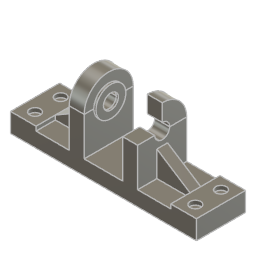
viking (Autodesk Fusion 360 design; units mm, degrees)
Autodesk Fusion 360 part; units mm, degrees
note: some values were not read from the file. Set by a fixed rule: which sketch regions a step uses.
sketch "Sketch1" plane through (0, 0, 0) normal (0, 1, 0) x (1, 0, 0)
  line L0 (0, 0) -> (87, 0)
  line L1 (0, 0) -> (-87, 0)
  line L2 (-87, 0) -> (-87, 46)
  line L3 (87, 0) -> (87, 46)
  line L4 (-87, 46) -> (87, 46)
  dimension "d1" = 87
  dimension "d2" = 87
  dimension "d3" = 46
  dimension "d4" = 46
  constraint coincident L0.start L1.start
  constraint horizontal L0
  constraint parallel L0 L1
  constraint perpendicular L1 L2
  constraint perpendicular L0 L3
  measures "d1" distance of L0.start L0.end
  measures "d2" distance of L0.start L1.end
  measures "d3" distance of L1.end L2.end
  measures "d4" distance of L0.end L3.end
extrude "Extrude1" add sketch "Sketch1" along normal blind 14 makes body 1
sketch "Sketch2" plane through (0, 14, 0) normal (0, 1, 0) x (-1, 0, 0)
  line L0 (87, 0) -> (-87, 0)
  line L1 (-87, 0) -> (-87, -46)
  line L2 (-87, -46) -> (87, -46)
  line L3 (87, -46) -> (87, 0)
  line L4 (87, -46) -> (-87, -46)
  line L5 (-87, -46) -> (-87, 0)
  line L6 (-87, 0) -> (87, 0)
  line L7 (87, 0) -> (87, -46)
  line L8 (-87, -46) -> (-63, -46)
  line L9 (-63, -46) -> (-63, 0)
  line L10 (-63, 0) -> (-87, 0)
  line L11 (-87, 0) -> (-87, -46)
  line L12 (87, -46) -> (63, -46)
  line L13 (63, -46) -> (63, 0)
  line L14 (63, 0) -> (87, 0)
  line L15 (87, 0) -> (87, -46)
  line L16 (87, -46) -> (87, -23) construction
  line L17 (87, -23) -> (-87, -23) construction
  line L18 (87, -23) -> (87, -11) construction
  line L19 (87, -23) -> (87, -35) construction
  line L20 (87, -35) -> (-87, -35) construction
  line L21 (87, -11) -> (-87, -11) construction
  line L22 (87, -46) -> (75, -46) construction
  line L23 (75, -46) -> (75, 0) construction
  line L24 (-63, -46) -> (-75, -46) construction
  line L25 (-75, -46) -> (-75, 0) construction
  circle A0 centre (75, -35) radius 5
  circle A1 centre (75, -11) radius 5
  circle A2 centre (-75, -35) radius 5
  circle A3 centre (-75, -11) radius 5
  dimension "d7" = 24
  dimension "d8" = 24
  dimension "d9" = 46
  dimension "d10" = 12
  dimension "d11" = 12
  dimension "d12" = 10
  dimension "d13" = 10
  dimension "d14" = 10
  dimension "d15" = 10
  constraint horizontal L4
  constraint vertical L5
  constraint horizontal L6
  constraint vertical L7
  constraint coincident L0.end L1.start
  constraint coincident L2.end L3.start
  constraint horizontal L8
  constraint vertical L9
  constraint horizontal L10
  constraint vertical L11
  constraint coincident L6 L9.end
  constraint coincident L1.end L2.start
  constraint horizontal L12
  constraint vertical L13
  constraint horizontal L14
  constraint vertical L15
  constraint midpoint L3 L16.end
  constraint midpoint L11 L17.end
  constraint perpendicular L17 L18
  constraint perpendicular L17 L19
  constraint coincident L5 L20.end
  constraint perpendicular L5 L20
  constraint coincident L1 L21.end
  constraint perpendicular L1 L21
  constraint midpoint L12 L22.end
  constraint midpoint L14 L23.end
  constraint midpoint L8 L24.end
  constraint midpoint L10 L25.end
  constraint coincident L20 A0.centre
  constraint coincident L23 A0.centre
  constraint coincident L21 A1.centre
  constraint coincident L23 A1.centre
  constraint coincident L25 A2.centre
  constraint coincident L20 A2.centre
  constraint coincident L21 A3.centre
  constraint coincident L25 A3.centre
  measures "d7" distance of L1.end L8.end
  measures "d8" distance of L2.end L12.end
  measures "d9" distance of L2.end L0.start
  measures "d10" distance of L16.end L18.end
  measures "d11" distance of L16.end L19.end
  measures "d12" diameter of A0
  measures "d13" diameter of A1
  measures "d14" diameter of A2
  measures "d15" diameter of A3
extrude "Extrude2" add sketch "Sketch2" along normal blind 4 contours L0 L2 L3 L4 L6 L7 L12 L13 L14 L15 bodies 1
extrude "Extrude3" add sketch "Sketch2" along normal blind 4 contours L0 L1 L2 L4 L5 L6 L8 L9 L10 L11 bodies 1
sketch "Sketch3" plane through (0, 0, 0) normal (0, 0, 1) x (1, 0, 0)
  line L0 (-87, 0) -> (87, 0)
  line L1 (87, 0) -> (87, 18)
  line L2 (87, 18) -> (63, 18)
  line L3 (63, 18) -> (63, 14)
  line L4 (63, 14) -> (-63, 14)
  line L5 (-63, 14) -> (-63, 18)
  line L6 (-63, 18) -> (-87, 18)
  line L7 (-87, 18) -> (-87, 0)
  line L8 (0, 0) -> (-75, 0) construction
  line L9 (-75, 0) -> (-75, 18) construction
  line L10 (75, 18) -> (75, 0) construction
  line L11 (75, 0) -> (-75, 0) construction
  line L12 (87, 0) -> (32, 0) construction
  line L13 (0, 0) -> (75, 0) construction
  line L14 (32, 0) -> (32, 50) construction
  line L15 (32, 14) -> (32, 50)
  line L16 (32, 50) -> (18, 50)
  line L17 (18, 50) -> (18, 14)
  line L18 (32, 14) -> (-32, 14) construction
  line L19 (-32, 14) -> (-32, 50)
  line L20 (-32, 50) -> (-18, 50)
  line L21 (-18, 50) -> (-18, 14)
  dimension "d20" = 75
  dimension "d21" = 55
  dimension "d22" = 50
  dimension "d23" = 14
  dimension "d24" = 64
  dimension "d25" = 14
  constraint coincident L8.start L13.start
  constraint perpendicular L3 L8
  constraint midpoint L6 L9.end
  constraint coincident L0 L10.end
  constraint perpendicular L0 L10
  constraint coincident L0.end L1.start
  constraint perpendicular L1 L12
  constraint perpendicular L13 L14
  constraint coincident L4 L15.start
  constraint coincident L14 L15.start
  constraint perpendicular L14 L16
  constraint coincident L4 L17.end
  constraint perpendicular L4 L17
  constraint perpendicular L17 L18
  constraint perpendicular L18 L19
  constraint perpendicular L19 L20
  constraint coincident L18 L21.end
  measures "d20" distance of L8.start L8.end
  measures "d21" distance of L0.end L12.end
  measures "d22" distance of L12.end L14.end
  measures "d23" distance of L14.end L16.end
  measures "d24" distance of L15.start L18.end
  measures "d25" distance of L19.end L20.end
extrude "Extrude4" add sketch "Sketch3" against normal blind 46 contours L4 L15 L16 L17 bodies 1
extrude "Extrude5" add sketch "Sketch3" against normal blind 46 contours L4 L19 L20 L21 bodies 1
sketch "Sketch4" plane through (-18, 0, 0) normal (1, 0, 0) x (0, 0, -1)
  line L0 (0, 50) -> (0, 14)
  line L1 (0, 14) -> (46, 14)
  line L2 (46, 14) -> (46, 50)
  line L3 (46, 50) -> (0, 50)
  line L4 (0, 50) -> (0, 18)
  line L5 (0, 18) -> (46, 18)
  line L6 (46, 18) -> (46, 50)
  line L7 (46, 50) -> (0, 50)
  circle A0 centre (23, 50) radius 14
  circle A1 centre (23, 50) radius 7
  arc A2 (46, 50) -> (0, 50) centre (23, 50) ccw
  line L8 (0, 50) -> (0, 18)
  line L9 (0, 18) -> (46, 18)
  line L10 (46, 18) -> (46, 50)
  dimension "d30" = 28
  dimension "d31" = 14
  constraint coincident L0.start L3.end
  constraint coincident L0 L4.end
  constraint perpendicular L1 L4
  constraint coincident L2 L5.end
  constraint perpendicular L2 L5
  constraint coincident L2.end L3.start
  constraint perpendicular L3 L6
  constraint midpoint L7 A0.centre
  constraint coincident L2.end A2
  constraint concentric A0 A2
  constraint concentric A0 A1
  constraint perpendicular L5 L8
  measures "d30" diameter of A0
  measures "d31" diameter of A1
extrude "Extrude6" add sketch "Sketch4" against normal blind 14 contours L3 L7 A0 A2 bodies 1
extrude "Extrude7" add sketch "Sketch4" along normal blind 2 separate body contours L3 L7 A0 A1 picked at (29.4096, 59.7107) makes body 2
extrude "Extrude8" add sketch "Sketch4" along normal blind 2 contours L3 L7 A0 A1 picked at (11.4115, 48.9567) bodies 1 2
sketch "Sketch5" plane through (-32, 0, 0) normal (-1, 0, 0) x (0, 0, 1)
  line L0 (-9, 50) -> (-37, 50)
  arc A0 (-9, 50) -> (-37, 50) centre (-23, 50) ccw
  arc A1 (0, 50) -> (-46, 50) centre (-23, 50) ccw
  line L1 (-46, 50) -> (-46, 14)
  line L2 (-46, 14) -> (0, 14)
  line L3 (0, 14) -> (0, 50)
  circle A2 centre (-23, 50) radius 14
  circle A3 centre (-23, 50) radius 7
  arc A4 (0, 50) -> (-46, 50) centre (-23, 50) ccw
  dimension "d38" = 46
  dimension "d39" = 28
  dimension "d40" = 14
  constraint concentric A0 A4
  constraint concentric A2 A4
  constraint concentric A3 A4
  measures "d38" diameter of A4
  measures "d39" diameter of A2
  measures "d40" diameter of A3
extrude "Extrude9" add sketch "Sketch5" along normal blind 2 separate body contours L0 A2 A3 | L0 A0 A2 A3 makes body 3
sketch "Sketch6" plane through (32, 0, 0) normal (1, 0, 0) x (0, 0, -1)
  line L0 (0, 50) -> (0, 14)
  line L1 (0, 14) -> (46, 14)
  line L2 (46, 14) -> (46, 50)
  line L3 (46, 50) -> (0, 50)
  circle A0 centre (23, 50) radius 7
  line L4 (23, 57) -> (23, 73)
  line L5 (9, 50) -> (0, 50)
  line L6 (9, 50) -> (0, 50)
  arc A1 (46, 50) -> (0, 50) centre (23, 50) ccw
  dimension "d43" = 14
  dimension "d45" = 46
  constraint midpoint L3 A0.centre
  constraint concentric A0 A1
  constraint coincident A0 L4.start
  constraint coincident L4.end A1
  constraint vertical L4
  constraint coincident L3 L5.start
  constraint coincident L0.start L3.end
  measures "d43" diameter of A0
  measures "d45" diameter of A1
extrude "Extrude10" add sketch "Sketch6" against normal blind 14 separate body contours L3 A0 L4 A1 makes body 4
extrude "Extrude11" cut sketch "Sketch6" against normal blind 14 contours L3 A0 picked at (23.8525, 47.828) bodies 1
sketch "Sketch7" plane through (0, 0, 0) normal (0, 0, 1) x (1, 0, 0)
  line L0 (-87, 0) -> (87, 0)
  line L1 (87, 0) -> (87, 18)
  line L2 (87, 18) -> (63, 18)
  line L3 (63, 18) -> (63, 14)
  line L4 (63, 14) -> (32, 14)
  line L5 (32, 14) -> (32, 50)
  line L6 (32, 50) -> (18, 50)
  line L7 (18, 50) -> (18, 14)
  line L8 (18, 14) -> (-18, 14)
  line L9 (-18, 14) -> (-18, 50)
  line L10 (-18, 50) -> (-32, 50)
  line L11 (-32, 50) -> (-32, 14)
  line L12 (-32, 14) -> (-63, 14)
  line L13 (-63, 14) -> (-63, 18)
  line L14 (-63, 18) -> (-87, 18)
  line L15 (-87, 18) -> (-87, 0)
  line L16 (32, 50) -> (32, 38)
  line L17 (32, 38) -> (63, 18)
  line L18 (32, 38) -> (32, 14)
  line L19 (32, 14) -> (63, 14)
  line L20 (63, 14) -> (63, 10)
  line L21 (-32, 36) -> (-63, 18)
  line L22 (-63, 18) -> (-63, 14)
  line L23 (-63, 14) -> (-32, 14)
  line L24 (-32, 14) -> (-32, 36)
  dimension "d50" = 12
  constraint coincident L5.end L6.start
  constraint perpendicular L6 L16
  constraint coincident L2.end L3.start
  constraint coincident L4.end L5.start
  constraint coincident L3.end L4.start
  constraint perpendicular L2 L20
  constraint coincident L11 L21.start
  constraint coincident L13.end L14.start
  constraint coincident L12.end L13.start
  constraint coincident L11.end L12.start
  measures "d50" distance of L5.end L16.end
sketch "Sketch8" plane through (0, 0, -46) normal (0, 0, -1) x (-1, 0, 0)
  line L0 (-87, 0) -> (87, 0)
  line L1 (87, 0) -> (87, 18)
  line L2 (87, 18) -> (63, 18)
  line L3 (63, 18) -> (63, 14)
  line L4 (63, 14) -> (32, 14)
  line L5 (32, 14) -> (32, 50)
  line L6 (32, 50) -> (18, 50)
  line L7 (18, 50) -> (18, 14)
  line L8 (18, 14) -> (-18, 14)
  line L9 (-18, 14) -> (-18, 50)
  line L10 (-18, 50) -> (-32, 50)
  line L11 (-32, 50) -> (-32, 14)
  line L12 (-32, 14) -> (-63, 14)
  line L13 (-63, 14) -> (-63, 18)
  line L14 (-63, 18) -> (-87, 18)
  line L15 (-87, 18) -> (-87, 0)
  line L16 (-63, 18) -> (-32, 38)
  line L17 (-32, 38) -> (-32, 14)
  line L18 (-32, 14) -> (-63, 14)
  line L19 (63, 18) -> (32, 36)
  line L20 (32, 36) -> (32, 14)
  line L21 (32, 14) -> (63, 14)
  line L22 (63, 14) -> (63, 18)
  constraint coincident L13.end L14.start
  constraint coincident L11 L16.end
  constraint coincident L11.end L12.start
  constraint coincident L12.end L13.start
  constraint coincident L2.end L3.start
  constraint coincident L5 L19.end
  constraint coincident L4.end L5.start
  constraint coincident L3.end L4.start
extrude "Extrude12" add sketch "Sketch7" against normal blind 18 separate body contours L3 L4 L5 L17 L18 L19 makes body 5
extrude "Extrude13" add sketch "Sketch8" against normal blind 18 separate body contours L11 L12 L13 L16 L17 L18 makes body 6
extrude "Extrude14" add 1 faces at (42.3333, 23.3333, -18) along direction (0, 0, -1) blind 10 on bodies 5 bodies 1 3 4 5 6
sketch "Sketch9" plane through (0, 0, 0) normal (0, 0, 1) x (1, 0, 0)
  line L0 (-87, 0) -> (87, 0)
  line L1 (87, 0) -> (87, 18)
  line L2 (87, 18) -> (63, 18)
  line L3 (63, 18) -> (32, 38)
  line L4 (32, 38) -> (32, 50)
  line L5 (32, 50) -> (18, 50)
  line L6 (18, 50) -> (18, 14)
  line L7 (18, 14) -> (-18, 14)
  line L8 (-18, 14) -> (-18, 50)
  line L9 (-18, 50) -> (-32, 50)
  line L10 (-32, 50) -> (-32, 14)
  line L11 (-32, 14) -> (-63, 14)
  line L12 (-63, 14) -> (-63, 18)
  line L13 (-63, 18) -> (-87, 18)
  line L14 (-87, 18) -> (-87, 0)
  line L15 (32, 38) -> (32, 14)
  line L16 (32, 14) -> (63, 14)
  line L17 (63, 14) -> (63, 18)
  constraint coincident L3.end L4.start
  constraint parallel L4 L15
  constraint perpendicular L15 L16
  constraint coincident L2.end L3.start
extrude "Extrude15" cut sketch "Sketch9" against normal blind 18 contours L3 L15 L16 L17 bodies 1
sketch "Sketch10" plane through (0, 0, -46) normal (0, 0, -1) x (-1, 0, 0)
  line L0 (-87, 0) -> (87, 0)
  line L1 (87, 0) -> (87, 18)
  line L2 (87, 18) -> (63, 18)
  line L3 (63, 18) -> (63, 14)
  line L4 (63, 14) -> (32, 14)
  line L5 (32, 14) -> (32, 50)
  line L6 (32, 50) -> (18, 50)
  line L7 (18, 50) -> (18, 14)
  line L8 (18, 14) -> (-18, 14)
  line L9 (-18, 14) -> (-18, 50)
  line L10 (-18, 50) -> (-32, 50)
  line L11 (-32, 50) -> (-32, 38)
  line L12 (-32, 38) -> (-63, 18)
  line L13 (-63, 18) -> (-87, 18)
  line L14 (-87, 18) -> (-87, 0)
  line L15 (-63, 14) -> (-63, 18)
  line L16 (-63, 14) -> (-32, 14)
  line L17 (-32, 14) -> (-32, 39)
  line L18 (-63, 18) -> (-32, 38)
  constraint coincident L12.end L13.start
  constraint perpendicular L13 L15
  constraint perpendicular L9 L16
  constraint perpendicular L8 L17
  constraint coincident L11.end L12.start
extrude "Extrude16" cut sketch "Sketch10" against normal blind 18 contours L12 L15 L16 L17 L18 bodies 1
sketch "Sketch11" plane through (0, 0, 0) normal (0, 0, 1) x (1, 0, 0)
  line L0 (32, 14) -> (32, 50)
  line L1 (32, 50) -> (18, 50)
  line L2 (18, 50) -> (18, 14)
  line L3 (18, 14) -> (-18, 14)
  line L4 (-18, 14) -> (-18, 50)
  line L5 (-18, 50) -> (-32, 50)
  line L6 (-32, 50) -> (-32, 14)
  line L7 (-32, 14) -> (-63, 14)
  line L8 (-63, 14) -> (-63, 18)
  line L9 (-63, 18) -> (-87, 18)
  line L10 (-87, 18) -> (-87, 0)
  line L11 (-87, 0) -> (87, 0)
  line L12 (87, 0) -> (87, 18)
  line L13 (87, 18) -> (63, 18)
  line L14 (63, 18) -> (63, 14)
  line L15 (63, 14) -> (32, 14)
  line L16 (-63, 18) -> (-32, 36)
  line L17 (-32, 36) -> (-32, 14)
  line L18 (-32, 14) -> (-63, 14)
  line L19 (-63, 14) -> (-63, 18)
  constraint coincident L8.end L9.start
  constraint coincident L6 L16.end
  constraint coincident L6.end L7.start
  constraint coincident L7.end L8.start
sketch "Sketch12" plane through (0, 0, -46) normal (0, 0, -1) x (-1, 0, 0)
  line L0 (-63, 14) -> (-63, 18)
  line L1 (-63, 18) -> (-87, 18)
  line L2 (-87, 18) -> (-87, 0)
  line L3 (-87, 0) -> (87, 0)
  line L4 (87, 0) -> (87, 18)
  line L5 (87, 18) -> (63, 18)
  line L6 (63, 18) -> (63, 14)
  line L7 (63, 14) -> (32, 14)
  line L8 (32, 14) -> (32, 50)
  line L9 (32, 50) -> (18, 50)
  line L10 (18, 50) -> (18, 14)
  line L11 (18, 14) -> (-18, 14)
  line L12 (-18, 14) -> (-18, 50)
  line L13 (-18, 50) -> (-32, 50)
  line L14 (-32, 50) -> (-32, 14)
  line L15 (-32, 14) -> (-63, 14)
  line L16 (32, 36) -> (32, 14)
  line L17 (32, 14) -> (63, 14)
  line L18 (63, 18) -> (32, 36)
  constraint coincident L8 L16.start
  constraint coincident L7.end L8.start
  constraint coincident L6.end L7.start
  constraint coincident L5.end L6.start
extrude "Extrude17" add sketch "Sketch12" against normal blind 18 separate body contours L6 L7 L8 L16 L17 L18 makes body 7
extrude "Extrude18" add sketch "Sketch11" against normal blind 18 separate body contours L6 L7 L8 L16 L17 L18 L19 makes body 8
extrude "Extrude19" add 1 faces at (-42.3333, 22.6667, -28) along direction (0, 0, 1) blind 10 on bodies 7 bodies 1 4 7 3 8
sketch "Sketch13" plane through (0, 0, 0) normal (0, 0, 1) x (1, 0, 0)
  line L0 (32, 14) -> (32, 50)
  line L1 (32, 50) -> (18, 50)
  line L2 (18, 50) -> (18, 14)
  line L3 (18, 14) -> (-18, 14)
  line L4 (-18, 14) -> (-18, 50)
  line L5 (-18, 50) -> (-32, 50)
  line L6 (-32, 50) -> (-32, 36)
  line L7 (-32, 36) -> (-63, 18)
  line L8 (-63, 18) -> (-87, 18)
  line L9 (-87, 18) -> (-87, 0)
  line L10 (-87, 0) -> (87, 0)
  line L11 (87, 0) -> (87, 18)
  line L12 (87, 18) -> (63, 18)
  line L13 (63, 18) -> (63, 14)
  line L14 (63, 14) -> (32, 14)
  line L15 (-63, 18) -> (-63, 14)
  line L16 (-32, 36) -> (-32, 14)
  line L17 (-32, 14) -> (-63, 14)
  line L18 (-63, 18) -> (-32, 36)
  dimension "d67" = 4
  constraint coincident L7.end L8.start
  constraint perpendicular L8 L15
  constraint coincident L6.end L7.start
  constraint parallel L6 L16
  constraint perpendicular L15 L17
  measures "d67" distance of L7.end L15.end
sketch "Sketch14" plane through (0, 0, -46) normal (0, 0, -1) x (-1, 0, 0)
  line L0 (-63, 14) -> (-63, 18)
  line L1 (-63, 18) -> (-87, 18)
  line L2 (-87, 18) -> (-87, 0)
  line L3 (-87, 0) -> (87, 0)
  line L4 (87, 0) -> (87, 18)
  line L5 (87, 18) -> (63, 18)
  line L6 (63, 18) -> (32, 36)
  line L7 (32, 36) -> (32, 50)
  line L8 (32, 50) -> (18, 50)
  line L9 (18, 50) -> (18, 14)
  line L10 (18, 14) -> (-18, 14)
  line L11 (-18, 14) -> (-18, 50)
  line L12 (-18, 50) -> (-32, 50)
  line L13 (-32, 50) -> (-32, 14)
  line L14 (-32, 14) -> (-63, 14)
  line L15 (32, 36) -> (32, 14)
  line L16 (32, 14) -> (63, 14)
  line L17 (63, 14) -> (63, 18)
  constraint coincident L6.end L7.start
  constraint parallel L7 L15
  constraint perpendicular L15 L16
  constraint coincident L5.end L6.start
extrude "Extrude20" cut sketch "Sketch13" against normal blind 18 contours L7 L15 L16 L17 L18 bodies 1
extrude "Extrude21" cut sketch "Sketch14" against normal blind 18 contours L6 L15 L16 L17 bodies 1
extrude "Extrude22" cut 1 faces at (-18, 48.6398, -20.8717) along direction (-1, 0, 0) blind 12 on bodies 1 bodies 1
extrude "Extrude23" cut 1 faces at (-32, 46.7924, -23.9301) along direction (1, 0, 0) blind 435 on bodies 1 bodies 1
